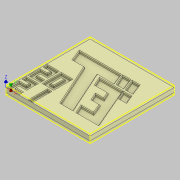
# Autodesk Inventor part: TestCAM
Saved by Autodesk Inventor 2021.2 (Build 252289000, 289)
## iProperties
Created: 2021-03-24
Part Number: TestCAM
Material: Generic
Document SubType Name: Modeling
Designer: Merkileg
Density: 1 g/cm^3
Appearance: Default
Author: Merkileg
Autodesk Inventor part; units mm, degrees
ref_plane "YZ Plane" through (0, 0, 0) normal (1, 0, 0) x (0, 1, 0)
ref_plane "XZ Plane" through (0, 0, 0) normal (0, 1, 0) x (-1, 0, 0)
ref_plane "XY Plane" through (0, 0, 0) normal (0, 0, 1) x (1, 0, 0)
sketch "Sketch1" plane through (0, 0, 0) normal (0, 1, 0) x (-1, 0, 0)
  line L0 (0, 0) -> (127, 0)
  line L1 (127, 0) -> (127, -127)
  line L2 (127, -127) -> (0, -127)
  line L3 (0, -127) -> (0, 0)
  dimension "d0" = 127
  dimension "d1" = 127
  constraints: 8 end point, 2 parallel, 1 horizontal, 1 perpendicular
  measures "d0" distance of L1.end L2.end
  measures "d1" distance of L0.end L1.end
extrude "Extrusion1" add sketch "Sketch1" along normal blind 6.35
sketch "Sketch2" plane through (0, 6.35, 0) normal (0, 1, 0) x (1, 0, 0)
  line L0 (-101.0761, 97.2689) -> (-28.5802, 97.2689) construction
  line L1 (-28.5802, 97.2689) -> (-28.5802, 40.6481) construction
  line L2 (-28.5802, 40.6481) -> (-101.0761, 40.6481) construction
  line L3 (-101.0761, 40.6481) -> (-101.0761, 97.2689) construction
  line L4 (0, 127) -> (-127, 127) construction
  line L5 (-63.5, 127) -> (-63.5, 0) construction
  line L6 (-127, 0) -> (0, 0) construction
  line L7 (0, 0) -> (0, 127) construction
  line L8 (0, 68.4911) -> (-127, 68.4911) construction
  line L9 (-127, 127) -> (-127, 0) construction
  point P0 (-63.5, 68.4911)
  constraints: 4 end point, 2 midpoint, 2 point on line, 1 perpendicular, 2 other
sketch "Sketch3" plane through (0, 6.35, 0) normal (0, 1, 0) x (1, 0, 0)
  line L0 (-119.2424, 103.5127) -> (-57.8091, 103.5127)
  line L1 (-57.8091, 103.5127) -> (-51.2894, 87.178)
  line L2 (-51.2894, 87.178) -> (-77.0149, 87.7134)
  line L3 (-77.0149, 87.7134) -> (-47.0419, 21.0184)
  line L4 (-47.0419, 21.0184) -> (-65.4412, 21.4013)
  line L5 (-65.4412, 21.4013) -> (-95.0024, 87.18)
  line L6 (-95.0024, 87.18) -> (-112.7234, 87.18)
  line L7 (-112.7234, 87.18) -> (-119.2424, 103.5127)
  line L8 (-54.1236, 103.8894) -> (-43.8878, 103.8894)
  line L9 (-43.8878, 103.8894) -> (-37.5996, 88.1349)
  line L10 (-37.5996, 88.1349) -> (-47.0419, 88.1349)
  line L11 (-47.0419, 88.1349) -> (-54.1236, 103.8894)
  line L12 (-39.9311, 103.8894) -> (-30.0436, 103.8894)
  line L13 (-30.0436, 103.8894) -> (-23.7555, 88.1349)
  line L14 (-23.7555, 88.1349) -> (-33.3468, 88.1349)
  line L15 (-33.3468, 88.1349) -> (-39.9311, 103.8894)
  line L16 (-68.2876, 83.1197) -> (-34.9034, 83.1197)
  line L17 (-34.9034, 83.1197) -> (-8.1984, 21.0184)
  line L18 (-8.1984, 21.0184) -> (-40.7437, 21.0184)
  line L19 (-40.7437, 21.0184) -> (-46.1306, 33.0052)
  line L20 (-46.1306, 33.0052) -> (-27.176, 33.1365)
  line L21 (-27.176, 33.1365) -> (-33.8867, 49.1932)
  line L22 (-33.8867, 49.1932) -> (-46.1306, 49.1932)
  line L23 (-46.1306, 49.1932) -> (-50.7359, 59.4408)
  line L24 (-50.7359, 59.4408) -> (-38.2057, 59.5276)
  line L25 (-38.2057, 59.5276) -> (-43.3076, 70.8801)
  line L26 (-43.3076, 70.8801) -> (-62.7871, 70.8801)
  line L27 (-62.7871, 70.8801) -> (-68.2876, 83.1197)
  line L28 (-31.9761, 83.1197) -> (-21.5509, 83.1197)
  line L29 (-21.5509, 83.1197) -> (-16.6151, 71.3098)
  line L30 (-16.6151, 71.3098) -> (-26.7635, 71.3098)
  line L31 (-26.7635, 71.3098) -> (-31.9761, 83.1197)
  point P0 (0, 0)
  constraints: 64 end point, 16 parallel, 5 point on line, 4 horizontal
extrude "Extrusion2" cut sketch "Sketch3" against normal blind 3.175
chamfer "Chamfer1" distance 1.0583 angle 45 32 edges at (-88.5257, 6.35, -103.5127) (-115.9829, 6.35, -95.3463) (-103.8629, 6.35, -87.18) (-80.2218, 6.35, -54.2906) (-56.2415, 6.35, -21.2099) (-62.0284, 6.35, -54.3659) (-64.1522, 6.35, -87.4457) (-54.5493, 6.35, -95.3454) (-50.5827, 6.35, -96.0122) (-49.0057, 6.35, -103.8894) (-40.7437, 6.35, -96.0122) (-42.3208, 6.35, -88.1349) (-36.6389, 6.35, -96.0122) (-34.9874, 6.35, -103.8894) (-26.8995, 6.35, -96.0122) (-28.5511, 6.35, -88.1349) (-26.7635, 6.35, -83.1197) (-29.3698, 6.35, -77.2147) (-21.6893, 6.35, -71.3098) (-19.083, 6.35, -77.2147) (-40.7567, 6.35, -65.2038) (-44.4708, 6.35, -59.4842) (-48.4333, 6.35, -54.317) (-40.0086, 6.35, -49.1932) (-30.5314, 6.35, -41.1648) (-36.6533, 6.35, -33.0708) (-43.4372, 6.35, -27.0118) (-24.471, 6.35, -21.0184) (-21.5509, 6.35, -52.069) (-51.5955, 6.35, -83.1197) (-65.5374, 6.35, -76.9999) (-53.0473, 6.35, -70.8801)
sketch "Sketch4" plane through (0, 6.35, 0) normal (0, 1, 0) x (1, 0, 0)
  line L0 (-124.7121, 60.5508) -> (-108.8371, 60.5508)
  line L1 (-108.8371, 60.5508) -> (-108.8371, 55.7955)
  line L2 (-108.8371, 55.7955) -> (-124.7121, 55.7955)
  line L3 (-124.7121, 55.7955) -> (-124.7121, 60.5508)
  line L4 (-108.8371, 60.5508) -> (-113.6166, 60.5508)
  line L5 (-113.6166, 60.5508) -> (-113.6166, 44.7)
  line L6 (-113.6166, 44.7) -> (-108.8371, 44.7)
  line L7 (-108.8371, 44.7) -> (-108.8371, 60.5508)
  line L8 (-108.8371, 44.7) -> (-124.7121, 44.7)
  line L9 (-124.7121, 44.7) -> (-124.7121, 49.4552)
  line L10 (-124.7121, 49.4552) -> (-108.8371, 49.4552)
  line L11 (-108.8371, 49.4552) -> (-108.8371, 44.7)
  line L12 (-124.7121, 49.4552) -> (-119.9569, 49.4552)
  line L13 (-119.9569, 49.4552) -> (-119.9569, 33.6044)
  line L14 (-119.9569, 33.6044) -> (-124.7121, 33.6044)
  line L15 (-124.7121, 33.6044) -> (-124.7121, 49.4552)
  line L16 (-124.7121, 33.6044) -> (-108.8371, 33.6044)
  line L17 (-108.8371, 33.6044) -> (-108.8371, 38.3596)
  line L18 (-108.8371, 38.3596) -> (-124.7121, 38.3596)
  line L19 (-124.7121, 38.3596) -> (-124.7121, 33.6044)
  line L20 (-104.1166, 60.5508) -> (-88.2658, 60.5508)
  line L21 (-88.2658, 60.5508) -> (-88.2658, 33.6044)
  line L22 (-88.2658, 33.6044) -> (-104.1166, 33.6044)
  line L23 (-104.1166, 33.6044) -> (-104.1166, 60.5508)
  line L24 (-99.3613, 55.7955) -> (-93.0367, 55.7955)
  line L25 (-93.0367, 55.7955) -> (-93.0367, 38.3596)
  line L26 (-93.0367, 38.3596) -> (-99.3613, 38.3596)
  line L27 (-99.3613, 38.3596) -> (-99.3613, 55.7955)
  line L28 (-124.7121, 28.8346) -> (-108.8371, 28.8346)
  line L29 (-108.8371, 28.8346) -> (-108.8371, 24.0794)
  line L30 (-108.8371, 24.0794) -> (-124.7121, 24.0794)
  line L31 (-124.7121, 24.0794) -> (-124.7121, 28.8346)
  line L32 (-108.8371, 28.8346) -> (-113.6166, 28.8346)
  line L33 (-113.6166, 28.8346) -> (-113.6166, 12.9838)
  line L34 (-113.6166, 12.9838) -> (-108.8371, 12.9838)
  line L35 (-108.8371, 12.9838) -> (-108.8371, 28.8346)
  line L36 (-108.8371, 12.9838) -> (-124.7121, 12.9838)
  line L37 (-124.7121, 12.9838) -> (-124.7121, 17.7391)
  line L38 (-124.7121, 17.7391) -> (-108.8371, 17.7391)
  line L39 (-108.8371, 17.7391) -> (-108.8371, 12.9838)
  line L40 (-124.7121, 17.7391) -> (-119.9569, 17.7391)
  line L41 (-119.9569, 17.7391) -> (-119.9569, 1.8882)
  line L42 (-119.9569, 1.8882) -> (-124.7121, 1.8882)
  line L43 (-124.7121, 1.8882) -> (-124.7121, 17.7391)
  line L44 (-124.7121, 1.8882) -> (-108.8371, 1.8882)
  line L45 (-108.8371, 1.8882) -> (-108.8371, 6.6435)
  line L46 (-108.8371, 6.6435) -> (-124.7121, 6.6435)
  line L47 (-124.7121, 6.6435) -> (-124.7121, 1.8882)
  line L48 (-93.021, 28.8346) -> (-88.2658, 28.8346)
  line L49 (-88.2658, 28.8346) -> (-88.2658, 1.8882)
  line L50 (-88.2658, 1.8882) -> (-93.021, 1.8882)
  line L51 (-93.021, 1.8882) -> (-93.021, 28.8346)
  point P0 (0, 0)
  point P1 (-124.7121, 22.4419)
  point P2 (-104.1166, 28.8346)
  point P3 (-99.3613, 28.8346)
  point P4 (-113.6166, 24.0794)
  point P5 (-113.6166, 17.7391)
  point P6 (-119.9569, 6.6435)
  point P7 (-119.9569, 12.9838)
  point P8 (-119.9569, 38.3596)
  point P9 (-119.9569, 44.7)
  point P10 (-113.6166, 44.7)
  point P11 (-113.6166, 55.7955)
  point P12 (-113.6166, 49.4552)
  dimension "d15" = 15.875
  dimension "d16" = 4.7552
  dimension "d17" = 4.7794
  dimension "d18" = 15.8508
  dimension "d19" = 4.7552
  dimension "d20" = 4.7552
  dimension "d21" = 15.8508
  dimension "d22" = 4.7552
  dimension "d26" = 6.3246
  dimension "d27" = 17.4359
  dimension "d28" = 15.875
  dimension "d29" = 4.7552
  dimension "d30" = 4.7794
  dimension "d31" = 15.8508
  dimension "d32" = 4.7552
  dimension "d33" = 4.7552
  dimension "d34" = 15.8508
  dimension "d35" = 4.7552
  constraints: 104 end point, 26 parallel, 13 horizontal, 13 perpendicular, 4 point on line
  measures "d15" distance of L1.end L2.end
  measures "d16" distance of L0.end L1.end
  measures "d17" distance of L6.end L5.end
  measures "d18" distance of L5.end L4.end
  measures "d19" distance of L8.end L9.end
  measures "d20" distance of L13.end L14.end
  measures "d21" distance of L12.end L13.end
  measures "d22" distance of L17.end L16.end
  measures "d26" distance of L25.end L26.end
  measures "d27" distance of L24.end L25.end
  measures "d28" distance of L30.start L30.end
  measures "d29" distance of L28.end L30.start
  measures "d30" distance of L34.end L34.start
  measures "d31" distance of L34.start L32.end
  measures "d32" distance of L37.start L40.start
  measures "d33" distance of L41.end L43.start
  measures "d34" distance of L40.end L41.end
  measures "d35" distance of L46.start L45.start
extrude "Extrusion3" cut sketch "Sketch4" against normal blind 3.175
chamfer "Chamfer2" distance 1.0583 angle 45 36 edges at (-124.7121, 6.35, -58.1732) (-116.7746, 6.35, -60.5508) (-119.1644, 6.35, -55.7955) (-113.6166, 6.35, -52.6254) (-119.1644, 6.35, -49.4552) (-124.7121, 6.35, -41.5298) (-116.7746, 6.35, -33.6044) (-108.8371, 6.35, -35.982) (-114.397, 6.35, -38.3596) (-119.9569, 6.35, -41.5298) (-114.397, 6.35, -44.7) (-108.8371, 6.35, -52.6254) (-99.3613, 6.35, -47.0776) (-96.199, 6.35, -55.7955) (-93.0367, 6.35, -47.0776) (-96.199, 6.35, -38.3596) (-96.1912, 6.35, -33.6044) (-88.2658, 6.35, -47.0776) (-96.1912, 6.35, -60.5508) (-104.1166, 6.35, -47.0776) (-124.7121, 6.35, -26.457) (-116.7746, 6.35, -28.8346) (-108.8371, 6.35, -20.9092) (-119.1644, 6.35, -24.0794) (-113.6166, 6.35, -20.9092) (-119.1644, 6.35, -17.7391) (-124.7121, 6.35, -9.8136) (-119.9569, 6.35, -9.8136) (-114.397, 6.35, -6.6435) (-116.7746, 6.35, -1.8882) (-108.8371, 6.35, -4.2659) (-114.397, 6.35, -12.9838) (-88.2658, 6.35, -15.3614) (-90.6434, 6.35, -28.8346) (-93.021, 6.35, -15.3614) (-90.6434, 6.35, -1.8882)
body "Solid1"
